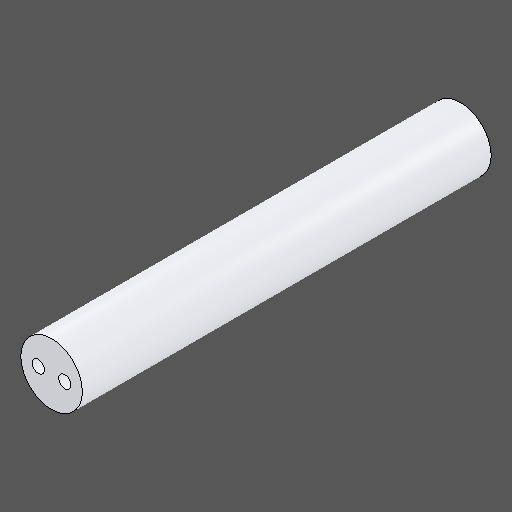
# Autodesk Inventor part: Ceramic-tube-two-holes-phi3x0.5
Saved by Autodesk Inventor 2025 (Build 290162000, 162)
## iProperties
Created: 2024-05-16
Part Number: Ceramic-tube-two-holes-phi3x0.5
Material: Polystyrene
Document SubType Name: Modeling
Designer: kuzmin
Density: 1.021 g/cm^3
Appearance: PTFE
Author: kuzmin
Autodesk Inventor part; units mm, degrees
ref_plane "YZ Plane" through (0, 0, 0) normal (1, 0, 0) x (0, 1, 0)
ref_plane "XZ Plane" through (0, 0, 0) normal (0, 1, 0) x (-1, 0, 0)
ref_plane "XY Plane" through (0, 0, 0) normal (0, 0, 1) x (1, 0, 0)
sketch "Sketch1" plane through (0, 0, 0) normal (0, 0, 1) x (1, 0, 0)
  circle A0 centre (-0.65, 0) radius 0.3
  circle A1 centre (0.65, 0) radius 0.3
  line L0 (-0.65, 0) -> (0.65, 0) construction
  circle A2 centre (0, 0) radius 1.5
  dimension "d4" = 0.6
  dimension "d5" = 1.3
  dimension "d6" = 3
  constraints: 3 centre point, 2 coincident, 2 end point, 1 equal radius, 1 horizontal, 1 midpoint
  measures "d4" diameter of A1
  measures "d5" distance of L0.start L0.end
  measures "d6" diameter of A2
extrude "Extrusion1" add sketch "Sketch1" along normal blind 20
body "Solid1"
